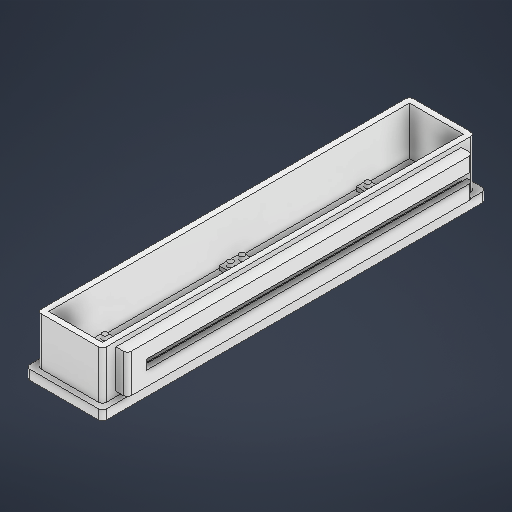
# Autodesk Inventor part: module_switch
Saved by Autodesk Inventor 2025.2 (Build 292293000, 293)
## iProperties
Created: 2025-09-07
Part Number: module_switch
Material: PC/ABS Plastic
Document SubType Name: Modeling
Designer: sam
Density: 1.1 g/cm^3
Appearance: Smooth - White
Author: sam
Autodesk Inventor part; units mm, degrees
ref_plane "YZ Plane" through (0, 0, 0) normal (1, 0, 0) x (0, 1, 0)
ref_plane "XZ Plane" through (0, 0, 0) normal (0, 1, 0) x (-1, 0, 0)
ref_plane "XY Plane" through (0, 0, 0) normal (0, 0, 1) x (1, 0, 0)
sketch "Sketch2" plane through (0, 0, 0) normal (0, 1, 0) x (-1, 0, 0)
  line L0 (-20, -100) -> (20, -100)
  line L1 (20, -100) -> (20, 100)
  line L2 (20, 100) -> (-20, 100)
  line L3 (-20, 100) -> (-20, -100)
  line L4 (-20, -100) -> (20, 100) construction
  line L5 (20, -100) -> (-20, 100) construction
  point P0 (0, 0)
  dimension "d0" = 40
  dimension "d1" = 200
  constraints: 12 end point, 2 midpoint, 2 parallel, 1 horizontal, 1 perpendicular
  measures "d0" distance of L2.end L1.end
  measures "d1" distance of L1.end L0.end
extrude "Extrusion1" add sketch "Sketch2" along normal blind 5
sketch "Sketch3" plane through (0, 5, 0) normal (0, 1, 0) x (1, 0, 0)
  line L0 (17, 97) -> (-17, 97)
  line L1 (-17, 97) -> (-17, -97)
  line L2 (-17, -97) -> (17, -97)
  line L3 (17, -97) -> (17, 97)
  line L4 (17, 97) -> (-17, -97) construction
  line L5 (-17, 97) -> (17, -97) construction
  line L6 (-20, 100) -> (-20, -100) projected
  line L7 (-20, -100) -> (20, -100) projected
  line L8 (14, 94) -> (-14, 94)
  line L9 (-14, 94) -> (-14, -94)
  line L10 (-14, -94) -> (14, -94)
  line L11 (14, -94) -> (14, 94)
  line L12 (14, 94) -> (-14, -94) construction
  line L13 (-14, 94) -> (14, -94) construction
  point P0 (0, 0)
  dimension "d4" = 3
  dimension "d5" = 3
  dimension "d6" = 3
  dimension "d7" = 3
  constraints: 24 end point, 4 midpoint, 4 parallel, 2 horizontal, 2 perpendicular
  measures "d4" distance between parallel lines of L6 L1
  measures "d5" distance between parallel lines of L7 L2
  measures "d6" distance between parallel lines of L2 L10
  measures "d7" distance between parallel lines of L1 L9
extrude "Extrusion2" add sketch "Sketch3" along normal blind 25
fillet "Fillet1" radius 2 8 edges at (17, 17.5, 97) (-17, 17.5, 97) (-20, 2.5, 100) (20, 2.5, 100) (17, 17.5, -97) (-17, 17.5, -97) (20, 2.5, -100) (-20, 2.5, -100)
sketch "Sketch4" plane through (17, 5, 95) normal (1, 0, 0) x (0, 0, -1)
  line L0 (5, 22.5) -> (185, 22.5)
  line L1 (185, 22.5) -> (185, 2.5)
  line L2 (185, 2.5) -> (5, 2.5)
  line L3 (5, 2.5) -> (5, 22.5)
  line L4 (190, 25) -> (190, 0) projected
  line L5 (0, 25) -> (190, 25) projected
  line L6 (0, 0) -> (0, 25) projected
  line L7 (190, 0) -> (0, 0) projected
  line L8 (-5, 0) -> (-5, -5) projected
  line L9 (195, -5) -> (195, 0) projected
  point P0 (95, -5)
  point P1 (0, 12.5)
  dimension "d42" = 10
  dimension "d43" = 10
  dimension "d44" = 20
  dimension "d45" = 10
  constraints: 8 end point, 2 parallel, 1 horizontal, 1 midpoint, 1 perpendicular
  measures "d42" distance between parallel lines of L8 L3
  measures "d43" distance between parallel lines of L9 L1
  measures "d44" distance between parallel lines of L0 L2
  measures "d45" distance from line of point (0, 12.5) L0
extrude "Extrusion3" add sketch "Sketch4" along normal blind 6 contours L0 L1 L2 L3
sketch "Sketch5" plane through (17, 7.5, -90) normal (0, 0, -1) x (-1, 0, 0)
  line L0 (0, 20) -> (0, 0) projected
  line L1 (0, 20) -> (-6, 20) projected
  line L2 (-6, 0) -> (-6, 20) projected
  line L3 (0, 0) -> (-6, 0) projected
  line L4 (-6, 12.5) -> (-3, 12.5)
  line L5 (-3, 12.5) -> (-3, 7.5)
  line L6 (-3, 7.5) -> (-6, 7.5)
  line L7 (-6, 7.5) -> (-6, 12.5)
  line L8 (0, 15) -> (-3, 15)
  line L9 (-3, 15) -> (-3, 5)
  line L10 (-3, 5) -> (0, 5)
  line L11 (0, 5) -> (0, 15)
  point P0 (17, -7.5)
  point P1 (-4.5, 7.5)
  point P2 (-4.5, 12.5)
  point P3 (-6, 7.5)
  point P4 (-3, 7.5)
  point P5 (0, 5)
  point P6 (-1.5, 15)
  dimension "d17" = 3
  dimension "d20" = 5
  dimension "d21" = 5
  dimension "d46" = 2.5
  dimension "d47" = 2.5
  constraints: 16 end point, 4 parallel, 3 midpoint, 3 point on line, 2 horizontal, 2 perpendicular
  measures "d17" distance of L5.end L6.end
  measures "d20" distance between parallel lines of L3 L10
  measures "d21" distance between parallel lines of L1 L8
  measures "d46" distance from line of L4 point (-1.5, 15)
  measures "d47" distance between parallel lines of L6 L10
extrude "Extrusion4" cut sketch "Sketch5" against normal blind 170 contours L0 L10 L9 L5 L8 | L4 L5 L6 L2
sketch "Sketch6" plane through (-17, 5, -95) normal (-1, 0, 0) x (0, 0, 1)
  line L0 (0, 0) -> (0, 25) projected
  line L1 (190, 0) -> (0, 0) projected
  line L2 (190, 25) -> (190, 0) projected
  line L3 (0, 25) -> (190, 25) projected
  line L4 (5, 17.5) -> (175, 17.5)
  line L5 (175, 17.5) -> (175, 7.5)
  line L6 (175, 7.5) -> (5, 7.5)
  line L7 (5, 7.5) -> (5, 17.5)
  line L8 (195, -5) -> (195, 0) projected
  line L9 (-5, 0) -> (-5, -5) projected
  point P0 (95, -5)
  point P1 (0, 12.5)
  dimension "d48" = 20
  dimension "d49" = 10
  dimension "d50" = 5
  dimension "d51" = 10
  constraints: 8 end point, 2 parallel, 1 horizontal, 1 midpoint, 1 perpendicular
  measures "d48" distance between parallel lines of L8 L5
  measures "d49" distance between parallel lines of L9 L7
  measures "d50" distance from line of point (0, 12.5) L4
  measures "d51" distance between parallel lines of L6 L4
extrude "Extrusion5" add sketch "Sketch6" along normal blind 6 contours L4 L5 L6 L7
sketch "Sketch7" plane through (-17, 12.5, 80) normal (0, 0, 1) x (1, 0, 0)
  line L0 (0, 10) -> (0, 0) projected
  line L1 (0, 10) -> (-6, 10) projected
  line L2 (-6, 0) -> (-6, 10) projected
  line L3 (0, 0) -> (-6, 0) projected
  line L4 (0, 10) -> (-3, 10)
  line L5 (-3, 10) -> (-3, 7.5)
  line L6 (-3, 7.5) -> (0, 7.5)
  line L7 (0, 7.5) -> (0, 10)
  line L8 (0, 0) -> (-3, 0)
  line L9 (-3, 0) -> (-3, 2.5)
  line L10 (-3, 2.5) -> (0, 2.5)
  line L11 (0, 2.5) -> (0, 0)
  point P0 (17, -12.5)
  dimension "d30" = 3
  dimension "d31" = 2.5
  dimension "d32" = 3
  dimension "d33" = 2.5
  constraints: 16 end point, 4 parallel, 2 horizontal, 2 perpendicular
  measures "d30" distance of L6.end L5.end
  measures "d31" distance of L5.end L4.end
  measures "d32" distance of L9.end L10.end
  measures "d33" distance of L8.end L9.end
extrude "Extrusion6" cut sketch "Sketch7" against normal up to surface (170 mm away) contours L0 L6 L5 L1 | L0 L3 L9 L10
fillet "Fillet3" radius 1 4 edges at (-18.5, 20, -90) (-18.5, 15, -90) (-18.5, 20, 80) (-18.5, 15, 80)
fillet "Fillet4" radius 1 4 edges at (-23, 22.5, -5) (-20, 22.5, -5) (-23, 12.5, -5) (-20, 12.5, -5)
fillet "Fillet5" radius 2 3 edges at (23, 17.5, 90) (23, 23.75, -90) (23, 11.25, -90)
fillet "Fillet6" radius 1 11 edges at (-22.7071, 22.2071, 80) (-21.5, 22.5, 80) (-20.2929, 22.2071, 80) (-20, 19.5, 80) (-20, 20.75, 80) (-22.7071, 12.7929, 80) (-21.5, 12.5, 80) (-20.2929, 12.7929, 80) (-20, 14.25, 80) (-20, 15.5, 80) (-23, 17.5, 80)
fillet "Fillet7" radius 1 11 edges at (-20.2929, 22.2071, -90) (-21.5, 22.5, -90) (-22.7071, 22.2071, -90) (-23, 17.5, -90) (-22.7071, 12.7929, -90) (-21.5, 12.5, -90) (-20.2929, 12.7929, -90) (-20, 15.5, -90) (-20, 14.25, -90) (-20, 20.75, -90) (-20, 19.5, -90)
sketch "Sketch8" plane through (0, 5, 0) normal (0, 1, 0) x (1, 0, 0)
  line L0 (14, 94) -> (-14, 94) projected
  line L1 (-14, 94) -> (-14, -94) projected
  line L2 (-14, -94) -> (14, -94) projected
  line L3 (14, -94) -> (14, 94) projected
  line L4 (12.75, 71) -> (-12.75, 71)
  line L5 (-12.75, 71) -> (-12.75, -71)
  line L6 (-12.75, -71) -> (12.75, -71)
  line L7 (12.75, -71) -> (12.75, 71)
  line L8 (12.75, 71) -> (-12.75, -71) construction
  line L9 (-12.75, 71) -> (12.75, -71) construction
  line L10 (-7.25, -65.5) -> (-13.25, -65.5)
  line L11 (-13.25, -65.5) -> (-13.25, -71.5)
  line L12 (-13.25, -71.5) -> (-7.25, -71.5)
  line L13 (-7.25, -71.5) -> (-7.25, -65.5)
  line L14 (-7.25, -65.5) -> (-13.25, -71.5) construction
  line L15 (-13.25, -65.5) -> (-7.25, -71.5) construction
  line L16 (-13.25, 71.5) -> (-7.25, 71.5)
  line L17 (-7.25, 71.5) -> (-7.25, 65.5)
  line L18 (-7.25, 65.5) -> (-13.25, 65.5)
  line L19 (-13.25, 65.5) -> (-13.25, 71.5)
  line L20 (-13.25, 71.5) -> (-7.25, 65.5) construction
  line L21 (-7.25, 71.5) -> (-13.25, 65.5) construction
  line L22 (13.25, 71.5) -> (7.25, 71.5)
  line L23 (7.25, 71.5) -> (7.25, 65.5)
  line L24 (7.25, 65.5) -> (13.25, 65.5)
  line L25 (13.25, 65.5) -> (13.25, 71.5)
  line L26 (13.25, 71.5) -> (7.25, 65.5) construction
  line L27 (7.25, 71.5) -> (13.25, 65.5) construction
  line L28 (13.25, -65.5) -> (7.25, -65.5)
  line L29 (7.25, -65.5) -> (7.25, -71.5)
  line L30 (7.25, -71.5) -> (13.25, -71.5)
  line L31 (13.25, -71.5) -> (13.25, -65.5)
  line L32 (13.25, -65.5) -> (7.25, -71.5) construction
  line L33 (7.25, -65.5) -> (13.25, -71.5) construction
  line L34 (-13.25, 6) -> (-7.25, 6)
  line L35 (-7.25, 6) -> (-7.25, -6)
  line L36 (-7.25, -6) -> (-13.25, -6)
  line L37 (-13.25, -6) -> (-13.25, 6)
  line L38 (-13.25, 6) -> (-7.25, -6) construction
  line L39 (-7.25, 6) -> (-13.25, -6) construction
  line L40 (13.25, 6) -> (7.25, 6)
  line L41 (7.25, 6) -> (7.25, -6)
  line L42 (7.25, -6) -> (13.25, -6)
  line L43 (13.25, -6) -> (13.25, 6)
  line L44 (13.25, 6) -> (7.25, -6) construction
  line L45 (7.25, 6) -> (13.25, -6) construction
  point P0 (0, 0)
  point P1 (-10.25, -68.5)
  point P2 (-10.25, 68.5)
  point P3 (10.25, 68.5)
  point P4 (10.25, -68.5)
  point P5 (-10.25, 0)
  point P6 (10.25, 0)
  dimension "d52" = 25.5
  dimension "d53" = 142
  dimension "d54" = 6
  dimension "d55" = 6
  dimension "d56" = 2.5
  dimension "d57" = 2.5
  dimension "d58" = 6
  dimension "d59" = 6
  dimension "d60" = 2.5
  dimension "d61" = 2.5
  dimension "d62" = 6
  dimension "d63" = 6
  dimension "d64" = 2.5
  dimension "d65" = 2.5
  dimension "d66" = 6
  dimension "d67" = 6
  dimension "d68" = 2.5
  dimension "d69" = 2.5
  dimension "d78" = 6
  dimension "d79" = 12
  dimension "d80" = 6
  dimension "d81" = 12
  dimension "d82" = 2.5
  dimension "d83" = 2.5
  constraints: 84 end point, 14 midpoint, 14 parallel, 7 horizontal, 7 perpendicular
  measures "d52" distance of L6.end L5.end
  measures "d53" distance of L5.end L4.end
  measures "d54" distance of L12.end L11.end
  measures "d55" distance of L11.end L10.end
  measures "d56" distance from line of L5 point (-10.25, -68.5)
  measures "d57" distance from line of L6 point (-10.25, -68.5)
  measures "d58" distance of L17.end L18.end
  measures "d59" distance of L16.end L17.end
  measures "d60" distance from line of L4 point (-10.25, 68.5)
  measures "d61" distance from line of L5 point (-10.25, 68.5)
  measures "d62" distance of L24.end L23.end
  measures "d63" distance of L23.end L22.end
  measures "d64" distance from line of L7 point (10.25, 68.5)
  measures "d65" distance from line of L4 point (10.25, 68.5)
  measures "d66" distance of L30.end L29.end
  measures "d67" distance of L29.end L28.end
  measures "d68" distance from line of L7 point (10.25, -68.5)
  measures "d69" distance from line of L6 point (10.25, -68.5)
  measures "d78" distance of L35.end L36.end
  measures "d79" distance of L34.end L35.end
  measures "d80" distance of L42.end L41.end
  measures "d81" distance of L41.end L40.end
  measures "d82" distance from line of L5 point (-10.25, 0)
  measures "d83" distance from line of L7 point (10.25, 0)
extrude "Extrusion7" add sketch "Sketch8" along normal blind 4 contours L7 L24 L23 L4 | L4 L23 L22 L25 L24 L7 | L17 L18 L5 L4 | L4 L5 L18 L19 L16 L17 | L40 L43 L42 L7 | L7 L42 L41 L40 | L28 L31 L30 L29 L6 L7 | L7 L6 L29 L28 | L34 L35 L36 L5 | L5 L36 L37 L34 | L10 L13 L6 L5 | L5 L6 L13 L12 L11 L10
sketch "Sketch9" plane through (0, 9, 0) normal (0, 1, 0) x (1, 0, 0)
  line L0 (-13.25, 71.5) -> (-13.25, 65.5) projected
  line L1 (-13.25, 65.5) -> (-7.25, 65.5) projected
  line L2 (-7.25, 65.5) -> (-7.25, 71.5) projected
  line L3 (-7.25, 71.5) -> (-13.25, 71.5) projected
  line L4 (7.25, 71.5) -> (7.25, 65.5) projected
  line L5 (7.25, 65.5) -> (13.25, 65.5) projected
  line L6 (13.25, 65.5) -> (13.25, 71.5) projected
  line L7 (13.25, 71.5) -> (7.25, 71.5) projected
  line L8 (13.25, -65.5) -> (7.25, -65.5) projected
  line L9 (7.25, -65.5) -> (7.25, -71.5) projected
  line L10 (7.25, -71.5) -> (13.25, -71.5) projected
  line L11 (13.25, -71.5) -> (13.25, -65.5) projected
  line L12 (-7.25, -71.5) -> (-7.25, -65.5) projected
  line L13 (-7.25, -65.5) -> (-13.25, -65.5) projected
  line L14 (-13.25, -65.5) -> (-13.25, -71.5) projected
  line L15 (-13.25, -71.5) -> (-7.25, -71.5) projected
  circle A0 centre (-10.25, 68.5) radius 1.5
  circle A1 centre (10.25, 68.5) radius 1.5
  circle A2 centre (10.25, -68.5) radius 1.5
  circle A3 centre (-10.25, -68.5) radius 1.5
  circle A4 centre (-10.25, 3) radius 1.5
  line L16 (-7.25, 6) -> (-13.25, 6) projected
  circle A5 centre (10.25, 3) radius 1.5
  circle A6 centre (-10.25, -3) radius 1.5
  line L17 (-13.25, -6) -> (-7.25, -6) projected
  circle A7 centre (10.25, -3) radius 1.5
  line L18 (-7.25, 6) -> (-13.25, 6) projected
  line L19 (-13.25, 6) -> (-13.25, -6) projected
  line L20 (-13.25, -6) -> (-7.25, -6) projected
  line L21 (-7.25, -6) -> (-7.25, 6) projected
  line L22 (7.25, -6) -> (13.25, -6) projected
  line L23 (13.25, -6) -> (13.25, 6) projected
  line L24 (13.25, 6) -> (7.25, 6) projected
  line L25 (7.25, 6) -> (7.25, -6) projected
  point P0 (0, 0)
  dimension "d72" = 3
  dimension "d73" = 3
  dimension "d74" = 3
  dimension "d75" = 3
  dimension "d84" = 3
  dimension "d85" = 3
  dimension "d86" = 3
  dimension "d87" = 3
  dimension "d88" = 3
  dimension "d89" = 3
  constraints: 8 centre point
  measures "d72" diameter of A0
  measures "d73" diameter of A1
  measures "d74" diameter of A2
  measures "d75" diameter of A3
  measures "d84" diameter of A4
  measures "d85" distance from line of L16 A4.centre
  measures "d86" diameter of A5
  measures "d87" diameter of A6
  measures "d88" distance from line of L17 A6.centre
  measures "d89" diameter of A7
extrude "Extrusion8" cut sketch "Sketch9" against normal blind 2
body "Solid1"
